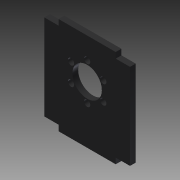
# Autodesk Inventor part: Motor Mount
Saved by Autodesk Inventor 2015 (Build 190159000, 159)
## iProperties
Created: 2016-09-19
Part Number: Motor Mount
Material: PVC, Unplasticized
Document SubType Name: Modeling
Designer: James Yelland
Density: 1.29 g/cm^3
Appearance: Smooth - White
Mass: 1.37738 g
Surface Area: 14.4739 cm^2
Volume: 1.06774 cm^3
Author: James Yelland
Autodesk Inventor part; units mm, degrees
ref_plane "YZ Plane" through (0, 0, 0) normal (1, 0, 0) x (0, 1, 0)
ref_plane "XZ Plane" through (0, 0, 0) normal (0, 1, 0) x (-1, 0, 0)
ref_plane "XY Plane" through (0, 0, 0) normal (0, 0, 1) x (1, 0, 0)
sketch "Sketch1" plane through (0, 0, 0) normal (0, 1, 0) x (-1, 0, 0)
  circle A0 centre (-5, 0.2) radius 5.15
  line L0 (10, -17.8) -> (10, 12.2)
  line L1 (-20, -17.8) -> (-20, 12.2)
  line L2 (10, 12.2) -> (5, 12.2)
  line L3 (5, 12.2) -> (5, 14.2)
  line L4 (-15, 14.2) -> (-15, 12.2)
  circle A1 centre (-5, 6.7) radius 1.1
  circle A2 centre (-10.6292, 3.45) radius 1.1
  circle A3 centre (-10.6292, -3.05) radius 1.1
  circle A4 centre (-5, -6.3) radius 1.1
  circle A5 centre (0.6292, -3.05) radius 1.1
  circle A6 centre (0.6292, 3.45) radius 1.1
  line L5 (-15, 12.2) -> (-20, 12.2)
  line L6 (5, 14.2) -> (-15, 14.2)
  line L7 (10, -17.8) -> (5, -17.8)
  line L8 (5, -17.8) -> (5, -19.8)
  line L9 (5, -19.8) -> (-15, -19.8)
  line L10 (-15, -19.8) -> (-15, -17.8)
  line L11 (-15, -17.8) -> (-20, -17.8)
  dimension "d7" = 360
  dimension "d42" = 30
  dimension "d43" = 5
  dimension "d44" = 2
  dimension "d49" = 2.2
  dimension "d52" = 360
  dimension "d54" = 10.3
  dimension "d57" = 30
  dimension "d58" = 15
  dimension "d59" = 5
  dimension "d60" = 2
  dimension "d61" = 20
  constraints: 24 end point, 7 centre point, 4 horizontal, 4 perpendicular, 3 vertical, 1 coincident, 1 point on line, 14 other
  measures "d42" distance of L1.start L1.end
  measures "d43" distance of L0.end L2.end
  measures "d44" distance of L2.end L3.end
  measures "d49" diameter of A1
  measures "d54" diameter of A0
  measures "d57" distance between parallel lines of L1 L0
  measures "d58" distance from line of L1 point (-5, 0.2)
  measures "d59" distance of L0.start L7.end
  measures "d60" distance of L7.end L8.end
  measures "d61" distance of L8.end L9.end
extrude "Extrusion1" add sketch "Sketch1" along normal blind 2
body "Solid1"
